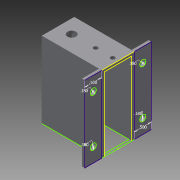
# Autodesk Inventor part: Autonomous - Ultrasonic Servo Mount V2
Saved by Autodesk Inventor 2015 (Build 190159000, 159)
## iProperties
Created: 2015-04-23
Part Number: Autonomous - Ultrasonic Servo Mount V2
Material: Generic
Document SubType Name: Modeling
Designer: WillHuie
Density: 1 g/cm^3
Appearance: Default
Author: WillHuie
Autodesk Inventor part; units mm, degrees
ref_plane "YZ Plane" through (0, 0, 0) normal (1, 0, 0) x (0, 1, 0)
ref_plane "XZ Plane" through (0, 0, 0) normal (0, 1, 0) x (-1, 0, 0)
ref_plane "XY Plane" through (0, 0, 0) normal (0, 0, 1) x (1, 0, 0)
sketch "Sketch1" plane through (0, 0, 0) normal (0, 1, 0) x (-1, 0, 0)
  line L0 (20.32, 10.16) -> (-20.32, 10.16)
  line L1 (-20.32, 10.16) -> (-20.32, -10.16)
  line L2 (-20.32, -10.16) -> (20.32, -10.16)
  line L3 (20.32, -10.16) -> (20.32, 10.16)
  line L4 (22.225, 12.065) -> (-22.225, 12.065)
  line L5 (-22.225, 12.065) -> (-22.225, -12.065)
  line L6 (-22.225, -12.065) -> (22.225, -12.065)
  line L7 (22.225, -12.065) -> (22.225, 12.065)
  point P0 (0, 0)
  dimension "d0" = 40.64
  dimension "d1" = 20.32
  dimension "d2" = 40.64
  dimension "d3" = 44.45
  dimension "d4" = 24.13
  dimension "d5" = 44.45
  constraints: 16 end point, 3 perpendicular, 2 parallel, 1 horizontal
  measures "d0" distance of L0.start L0.end
  measures "d1" distance of L0.end L1.end
  measures "d2" distance of L1.end L2.end
  measures "d3" distance of L4.start L4.end
  measures "d4" distance of L4.end L5.end
  measures "d5" distance of L5.end L6.end
extrude "Extrusion1" add sketch "Sketch1" along normal blind 56.515
sketch "Sketch2" plane through (-20.32, 0, -10.16) normal (1, 0, 0) x (0, 0, -1)
  line L0 (0, 0) -> (-20.32, 0) projected
  line L1 (0, 0) -> (0, 56.515) projected
  line L2 (-20.32, 56.515) -> (0, 56.515) projected
  line L3 (-20.32, 0) -> (-20.32, 56.515) projected
  point P0 (-10.16, 0)
extrude "Extrusion2" cut sketch "Sketch2" against normal blind 56.515
sketch "Sketch3" plane through (20.32, 0, 10.16) normal (-1, 0, 0) x (0, 0, 1)
  line L0 (0, 0) -> (-20.32, 0) projected
  line L1 (0, 0) -> (0, 56.515) projected
  line L2 (-20.32, 56.515) -> (0, 56.515) projected
  line L3 (-20.32, 0) -> (-20.32, 56.515) projected
  point P0 (-10.16, 0)
extrude "Extrusion3" cut sketch "Sketch3" against normal blind 56.515
sketch "Sketch4" plane through (22.225, 0, 10.16) normal (0, 0, -1) x (-1, 0, 0)
  line L0 (44.45, 56.515) -> (44.45, 0) projected
  line L1 (0, 56.515) -> (44.45, 56.515) projected
  line L2 (0, 0) -> (0, 56.515) projected
  line L3 (44.45, 54.61) -> (0, 54.61)
  point P0 (22.225, 0)
  constraints: 2 end point, 2 point on line, 1 perpendicular
extrude "Extrusion4" add sketch "Sketch4" along normal blind 20.32
sketch "Sketch7" plane through (0, 56.515, 0) normal (0, 1, 0) x (1, 0, 0)
  circle A0 centre (18.415, 0) radius 1.5875
  circle A1 centre (5.715, 0) radius 1.5875
  circle A2 centre (-12.065, 0) radius 3.175
  point P0 (0, 0)
  dimension "d18" = 3.175
  dimension "d19" = 3.175
  dimension "d20" = 6.35
  constraints: 3 centre point
  measures "d18" diameter of A0
  measures "d19" diameter of A1
  measures "d20" diameter of A2
extrude "Extrusion7" cut sketch "Sketch7" against normal blind 15.24
sketch "Sketch10" plane through (0, 56.515, 0) normal (0, 1, 0) x (1, 0, 0)
  circle A0 centre (-12.065, 0) radius 3.175 projected
  line L0 (-22.225, 12.065) -> (-22.225, -12.065) projected
  line L1 (-22.225, -12.065) -> (22.225, -12.065) projected
  line L2 (22.225, 12.065) -> (-22.225, 12.065) projected
  line L3 (1.905, 12.065) -> (1.905, -12.065)
  point P0 (0, 0)
  constraints: 2 end point, 2 point on line, 1 perpendicular
extrude "Extrusion10" cut sketch "Sketch10" along normal blind 19.05
sketch "Sketch11" plane through (22.225, 0, 10.16) normal (1, 0, 0) x (0, 0, -1)
  line L0 (0, 0) -> (0, 54.61) projected
  line L1 (0, 54.61) -> (20.32, 54.61) projected
  line L2 (20.32, 54.61) -> (20.32, 0) projected
  line L3 (20.32, 0) -> (22.225, 0) projected
  line L4 (22.225, 0) -> (22.225, 56.515) projected
  line L5 (-1.905, 56.515) -> (22.225, 56.515) projected
  line L6 (-1.905, 0) -> (-1.905, 56.515) projected
  line L7 (-1.905, 0) -> (0, 0) projected
  line L8 (-1.905, 0) -> (-1.905, 56.515)
  line L9 (-1.905, 56.515) -> (-14.605, 56.515)
  line L10 (-14.605, 56.515) -> (-14.605, 0)
  line L11 (-14.605, 0) -> (-1.905, 0)
  line L12 (22.225, 0) -> (34.925, 0)
  line L13 (34.925, 0) -> (34.925, 56.515)
  line L14 (34.925, 56.515) -> (22.225, 56.515)
  line L15 (22.225, 0) -> (22.225, 56.515)
  line L16 (22.225, 0) -> (22.225, 56.515) projected
  line L17 (-14.605, 56.515) -> (-8.255, 56.515)
  circle A0 centre (-8.255, 10.5386) radius 2.286
  circle A1 centre (-8.255, 45.974) radius 2.286
  circle A2 centre (28.575, 45.974) radius 2.286
  circle A3 centre (28.575, 10.5386) radius 2.286
  point P0 (10.16, 0)
  dimension "d38" = 12.7
  dimension "d39" = 12.7
  dimension "d42" = 4.572
  dimension "d44" = 4.572
  dimension "d45" = 4.572
  dimension "d46" = 4.572
  constraints: 18 end point, 5 perpendicular, 4 centre point, 2 point on line, 1 collinear, 1 midpoint, 1 vertical
  measures "d38" distance of L5.start L9.end
  measures "d39" distance of L3.end L12.end
  measures "d42" diameter of A0
  measures "d44" diameter of A1
  measures "d45" diameter of A2
  measures "d46" diameter of A3
extrude "Extrusion11" add sketch "Sketch11" against normal blind 1.905 contours L11 L10 L9 L6 | L14 L13 L12 L4 | A0 | A1 | A2 | A3
extrude "Extrusion12" cut sketch "Sketch11" against normal blind 6.35 contours A0 | A1 | A2 | A3
body "Solid1"
